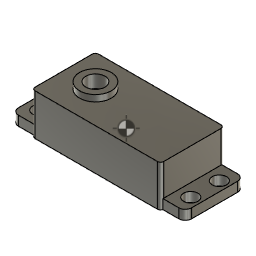
MG996R_Shell_Top v6 (Autodesk Fusion 360 design; units mm, degrees)
Autodesk Fusion 360 part; units mm, degrees
sketch "Sketch1" plane through (0, 0, 0) normal (0, 0, 1) x (1, 0, 0)
  line L0 (-19.8608, 0) -> (46.1392, 0) construction
  line L1 (-17, -9.25) -> (-10, -9.25)
  line L2 (-10, -9.25) -> (-10, -10)
  line L3 (-10, -10) -> (30.5, -10)
  line L4 (30.5, -10) -> (30.5, -9.25)
  line L5 (30.5, -9.25) -> (37.5, -9.25)
  line L6 (37.5, -9.25) -> (37.5, 0)
  circle A0 centre (-13, -4.5) radius 2.25
  line L7 (-17, -9.25) -> (-17, 0)
  circle A1 centre (34.5, -4.5) radius 2.25
  line L8 (30.5, 10) -> (30.5, 9.25)
  line L9 (-10, 9.25) -> (-10, 10)
  line L10 (-17, 9.25) -> (-17, 0)
  line L11 (37.5, 9.25) -> (37.5, 0)
  line L12 (30.5, 9.25) -> (37.5, 9.25)
  circle A2 centre (-13, 4.5) radius 2.25
  line L13 (-10, 10) -> (30.5, 10)
  line L14 (-17, 9.25) -> (-10, 9.25)
  circle A3 centre (34.5, 4.5) radius 2.25
  point P0 (46.1392, 0)
  point P1 (-19.8608, 0)
  dimension "d1" = 4.5
  dimension "d2" = 10
  dimension "d3" = 4.5
  dimension "d4" = 47.5
  dimension "d5" = 7
  dimension "d6" = 7
  dimension "d7" = 4
  dimension "d8" = 4
  dimension "d9" = 4.5
  dimension "d10" = 4.5
  dimension "d11" = 10
  dimension "d12" = 10
  dimension "d13" = 9.25
  dimension "d14" = 9.25
  constraint horizontal L0
  constraint perpendicular L1 L2
  constraint perpendicular L3 L4
  constraint perpendicular L4 L5
  constraint coincident L0 L6.end
  constraint perpendicular L0 L6
  constraint coincident L0 L7.end
  constraint perpendicular L0 L7
  constraint coincident origin L0
  constraint symmetric P1 L0 L0.start
  constraint symmetric P0 L0 L0.end
  constraint symmetric L0 L1.start L10.start
  constraint symmetric L0 L1.end L9.start
  constraint symmetric L0 L2.end L9.end
  constraint symmetric L0 L3.end L8.start
  constraint symmetric L0 L4.end L8.end
  constraint symmetric L0 L5.end L11.start
  constraint symmetric L0 L6.end L11.end
  constraint symmetric L0 A0 A2
  constraint symmetric L0 L7.end L10.end
  constraint symmetric L0 A1 A3
  measures "d1" diameter of A1
  measures "d2" distance of L0 L3
  measures "d3" distance of L0 A1.centre
  measures "d4" horizontal distance of A0.centre A1.centre
  measures "d5" distance of L2 L7
  measures "d6" distance of L4 L6
  measures "d7" distance of L4 A1.centre
  measures "d8" distance of A0.centre L7
  measures "d9" diameter of A0
  measures "d10" distance of L0 A0.centre
  measures "d11" distance of origin L2
  measures "d12" distance of L0 L3
  measures "d13" distance of L0 L1
  measures "d14" distance of L0 L5
extrude "Extrude1" add sketch "Sketch1" along normal blind 13
sketch "Sketch3" plane through (0, -9.25, 0) normal (0, -1, 0) x (1, 0, 0)
  line L0 (30.5, 0) -> (37.5, 0)
  line L1 (37.5, 0) -> (37.5, 13)
  line L2 (37.5, 13) -> (30.5, 13)
  line L3 (30.5, 13) -> (30.5, 0)
  line L4 (37.5, 0) -> (30.5, 0)
  line L5 (30.5, 0) -> (30.5, 3)
  line L6 (30.5, 3) -> (37.5, 3)
  line L7 (37.5, 3) -> (37.5, 0)
  line L8 (-10, 0) -> (-17, 0)
  line L9 (-17, 0) -> (-17, 3)
  line L10 (-17, 3) -> (-10, 3)
  line L11 (-10, 3) -> (-10, 0)
  dimension "d21" = 3
  dimension "d22" = 3
  constraint horizontal L4
  constraint vertical L5
  constraint horizontal L6
  constraint vertical L7
  constraint coincident L3 L5.end
  constraint coincident L0.end L1.start
  constraint horizontal L8
  constraint vertical L9
  constraint horizontal L10
  constraint vertical L11
  measures "d21" distance of L8.start L10.end
  measures "d22" distance of L0.start L5.end
extrude "Extrude3" cut sketch "Sketch3" against normal blind 26 contours L1 L2 L3 L6
sketch "Sketch4" plane through (0, -9.25, 0) normal (0, -1, 0) x (1, 0, 0)
  line L0 (-17, 0) -> (-10, 0)
  line L1 (-10, 0) -> (-10, 13)
  line L2 (-10, 13) -> (-17, 13)
  line L3 (-17, 13) -> (-17, 0)
  line L4 (-17, 0) -> (-10, 0)
  line L5 (-10, 0) -> (-10, 3)
  line L6 (-10, 3) -> (-17, 3)
  line L7 (-17, 3) -> (-17, 0)
  dimension "d25" = 3
  constraint horizontal L4
  constraint vertical L5
  constraint horizontal L6
  constraint vertical L7
  constraint coincident L1 L5.end
  constraint coincident L0.start L3.end
  measures "d25" distance of L0.start L6.end
extrude "Extrude4" cut sketch "Sketch4" against normal blind 22 contours L1 L2 L3 L6
sketch "Sketch5" plane through (0, 0, 13) normal (0, 0, 1) x (-1, 0, 0)
  line L0 (10, -10) -> (10, 10)
  line L1 (10, 10) -> (-30.5, 10)
  line L2 (-30.5, 10) -> (-30.5, -10)
  line L3 (-30.5, -10) -> (10, -10)
  circle A0 centre (0, 0) radius 3
  dimension "d28" = 6
  constraint coincident A0.centre origin
  measures "d28" diameter of A0
extrude "Extrude5" cut sketch "Sketch5" against normal blind 21 contours A0
sketch "Sketch6" plane through (0, 0, 0) normal (0, 0, -1) x (-1, 0, 0)
  circle A0 centre (0, 0) radius 3
  line L0 (10, -10) -> (10, 10)
  line L1 (10, 10) -> (-33, 10)
  line L2 (-33, 10) -> (-33, -10)
  line L3 (-33, -10) -> (10, -10)
  circle A1 centre (-11, 0) radius 0.75
  circle A2 centre (-20.5, 0) radius 0.75
  circle A3 centre (0, 0) radius 3
  circle A4 centre (-34.5, 4.5) radius 2.25
  circle A5 centre (13, -4.5) radius 2.25
  circle A6 centre (-34.5, -4.5) radius 2.25
  circle A7 centre (13, 4.5) radius 2.25
  line L4 (10, -9.25) -> (17, -9.25)
  line L5 (17, -9.25) -> (17, 9.25)
  line L6 (17, 9.25) -> (10, 9.25)
  line L7 (10, 9.25) -> (10, 10)
  line L8 (10, 10) -> (-30.5, 10)
  line L9 (-30.5, 10) -> (-30.5, 9.25)
  line L10 (-30.5, 9.25) -> (-37.5, 9.25)
  line L11 (-37.5, 9.25) -> (-37.5, -9.25)
  line L12 (-37.5, -9.25) -> (-30.5, -9.25)
  line L13 (-30.5, -9.25) -> (-30.5, -10)
  line L14 (-30.5, -10) -> (10, -10)
  line L15 (10, -10) -> (10, -9.25)
  dimension "d31" = 1.5
  dimension "d32" = 1.5
  dimension "d33" = 11
  dimension "d34" = 9.5
  measures "d31" diameter of A1
  measures "d32" diameter of A2
  measures "d33" distance of A0.centre A1.centre
  measures "d34" distance of A1.centre A2.centre
extrude "Extrude6" cut sketch "Sketch6" against normal blind 12 contours A1 | A2
sketch "Sketch7" plane through (0, 0, 0) normal (0, 0, -1) x (1, 0, 0)
  circle A0 centre (11, 0) radius 0.75
  circle A1 centre (20.5, 0) radius 0.75
  circle A2 centre (0, 0) radius 3
  circle A3 centre (34.5, -4.5) radius 2.25
  circle A4 centre (-13, 4.5) radius 2.25
  circle A5 centre (34.5, 4.5) radius 2.25
  circle A6 centre (-13, -4.5) radius 2.25
  line L0 (-10, 9.25) -> (-17, 9.25)
  line L1 (-17, 9.25) -> (-17, -9.25)
  line L2 (-17, -9.25) -> (-10, -9.25)
  line L3 (-10, -9.25) -> (-10, -10)
  line L4 (-10, -10) -> (30.5, -10)
  line L5 (30.5, -10) -> (30.5, -9.25)
  line L6 (30.5, -9.25) -> (37.5, -9.25)
  line L7 (37.5, -9.25) -> (37.5, 9.25)
  line L8 (37.5, 9.25) -> (30.5, 9.25)
  line L9 (30.5, 9.25) -> (30.5, 10)
  line L10 (30.5, 10) -> (-10, 10)
  line L11 (-10, 10) -> (-10, 9.25)
  line L12 (29.5, 9) -> (-9, 9)
  line L13 (-9, 9) -> (-9, -9)
  line L14 (-9, -9) -> (29.5, -9)
  line L15 (29.5, -9) -> (29.5, 9)
  line L16 (29.5, 9) -> (-9, -9) construction
  line L17 (-9, 9) -> (29.5, -9) construction
  point P0 (10.25, 0)
  dimension "d37" = 1
  dimension "d38" = 1
  dimension "d39" = 1
  dimension "d40" = 1
  constraint horizontal L12
  constraint perpendicular L12 L13
  constraint parallel L12 L14
  constraint parallel L13 L15
  constraint coincident L16 P0
  constraint coincident L17 P0
  measures "d37" distance of L10 L12
  measures "d38" distance of L4 L14
  measures "d39" distance of L5 L15
  measures "d40" distance of L11 L13
extrude "Extrude7" cut sketch "Sketch7" against normal blind 12 contours L12 L13 L14 L15
sketch "Sketch8" plane through (0, 0, 12) normal (0, 0, -1) x (1, 0, 0)
  circle A0 centre (0, 0) radius 3
  line L0 (29.5, -9) -> (29.5, 9)
  line L1 (29.5, 9) -> (-9, 9)
  line L2 (-9, 9) -> (-9, -9)
  line L3 (-9, -9) -> (29.5, -9)
  circle A1 centre (11, 0) radius 0.75
  circle A2 centre (20.5, 0) radius 0.75
  circle A3 centre (11, 0) radius 1.75
  circle A4 centre (20.5, 0) radius 1.75
  dimension "d43" = 1.5
  dimension "d44" = 1.5
  dimension "d45" = 9.5
  dimension "d46" = 11
  dimension "d47" = 3.5
  dimension "d48" = 3.5
  constraint concentric A1 A3
  constraint concentric A2 A4
  measures "d43" diameter of A1
  measures "d44" diameter of A2
  measures "d45" distance of A1.centre A2.centre
  measures "d46" distance of A0.centre A1.centre
  measures "d47" diameter of A3
  measures "d48" diameter of A4
extrude "Extrude8" add sketch "Sketch8" along normal blind 1 contours A3 | A4
sketch "Sketch9" plane through (0, 0, 12) normal (0, 0, -1) x (1, 0, 0)
  circle A0 centre (11, 0) radius 1.75
  circle A1 centre (0, 0) radius 3
  line L0 (29.5, -9) -> (29.5, 9)
  line L1 (29.5, 9) -> (-9, 9)
  line L2 (-9, 9) -> (-9, -9)
  line L3 (-9, -9) -> (29.5, -9)
  circle A2 centre (20.5, 0) radius 1.75
  circle A3 centre (0, 0) radius 3
  circle A4 centre (0, 0) radius 5
  dimension "d51" = 2
  constraint concentric A1 A3
  constraint concentric A3 A4
  measures "d51" distance of A3 A4
extrude "Extrude9" add sketch "Sketch9" along normal blind 1 contours A4
sketch "Sketch10" plane through (0, 0, 13) normal (0, 0, 1) x (-1, 0, 0)
  circle A0 centre (0, 0) radius 3
  line L0 (10, -10) -> (10, 10)
  line L1 (10, 10) -> (-30.5, 10)
  line L2 (-30.5, 10) -> (-30.5, -10)
  line L3 (-30.5, -10) -> (10, -10)
  circle A1 centre (0, 0) radius 3
  circle A2 centre (0, 0) radius 5
  dimension "d54" = 2
  constraint concentric A0 A1
  constraint concentric A1 A2
  measures "d54" distance of A1 A2
extrude "Extrude10" add sketch "Sketch10" along normal blind 2 contours A2
fillet "Fillet1" radius 1 4 edges at (30.5, -10, 6.5) (30.5, 10, 6.5) (-10, -10, 6.5) (-10, 10, 6.5)
fillet "Fillet2" radius 2 4 edges at (37.5, -9.25, 1.5) (37.5, 9.25, 1.5) (-17, -9.25, 1.5) (-17, 9.25, 1.5)
sketch "Sketch11" plane through (0, 0, 12) normal (0, 0, -1) x (1, 0, 0)
  circle A0 centre (0, 0) radius 5 construction
  circle A1 centre (11, 0) radius 1.75 construction
  line L0 (29.5, -9) -> (29.5, 9) construction
  line L1 (29.5, 9) -> (-9, 9) construction
  line L2 (-9, 9) -> (-9, -9) construction
  line L3 (-9, -9) -> (29.5, -9) construction
  circle A2 centre (20.5, 0) radius 1.75 construction
  line L4 (28.25, -7.5) -> (-7.75, -7.5) construction
  line L5 (-7.75, -7.5) -> (-7.75, 7.5) construction
  line L6 (-7.75, 7.5) -> (28.25, 7.5) construction
  line L7 (28.25, 7.5) -> (28.25, -7.5) construction
  circle A3 centre (-7.75, 7.5) radius 0.875
  circle A4 centre (-7.75, -7.5) radius 0.875
  circle A5 centre (28.25, 7.5) radius 0.875
  circle A6 centre (28.25, -7.5) radius 0.875
  circle A7 centre (28.25, 7.5) radius 1.875
  circle A8 centre (28.25, -7.5) radius 1.875
  circle A9 centre (-7.75, -7.5) radius 1.875
  circle A10 centre (-7.75, 7.5) radius 1.875
  line L8 (-9, 10) -> (29.5, 10)
  line L9 (-9, -10) -> (29.5, -10)
  dimension "d63" = 1.25
  dimension "d66" = 1.75
  dimension "d67" = 1
  dimension "d70" = 36
  dimension "d71" = 15
  dimension "d73" = 2.5
  dimension "d74" = 2.5
  dimension "d75" = 1.25
  dimension "d76" = 1.25
  constraint horizontal L4
  constraint vertical L5
  constraint horizontal L6
  constraint vertical L7
  constraint coincident L5.end L6.start
  constraint coincident L4.end L5.start
  constraint coincident L6.end L7.start
  constraint coincident L4.start L7.end
  constraint equal A5 A6
  constraint equal A3 A6
  constraint equal A3 A4
  constraint concentric A6 A8
  constraint concentric A4 A9
  constraint concentric A3 A10
  constraint equal A9 A10
  constraint equal A8 A9
  constraint equal A7 A8
  measures "d63" distance of L2 L5
  measures "d66" diameter of A5
  measures "d67" distance of A5 A7
  measures "d70" distance of L5.end L6.end
  measures "d71" distance of L4.start L6.end
  measures "d73" distance of L6 L8
  measures "d74" distance of L4 L9
  measures "d75" distance of L2 L5
  measures "d76" distance of L0 L7
extrude "Extrude11" add sketch "Sketch11" along normal blind 12
equation "d13 = ( 18.5 / 2 ) * 1 mm"
equation "d14 = ( 18.5 / 2 ) * 1 mm"
